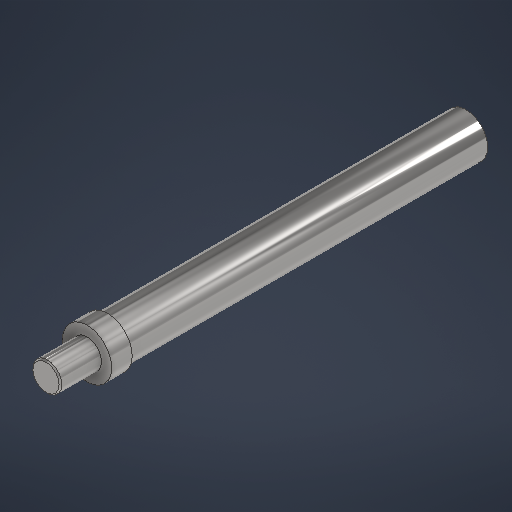
# Autodesk Inventor part: trục đai
Saved by Autodesk Inventor 2027.1 (Build 311270010, 270A)
## iProperties
Created: 2026-06-14
Part Number: trục đai
Material: Generic
Document SubType Name: Sheet Metal
Designer: MSI
Density: 1 g/cm^3
Sheet Metal Rule: Default_mm
Appearance: Steel - Polished
Author: MSI
Autodesk Inventor part; units mm, degrees
ref_plane "YZ Plane" through (0, 0, 0) normal (1, 0, 0) x (0, 1, 0)
ref_plane "XZ Plane" through (0, 0, 0) normal (0, 1, 0) x (-1, 0, 0)
ref_plane "XY Plane" through (0, 0, 0) normal (0, 0, 1) x (1, 0, 0)
sketch "Sketch1" plane through (0, 0, 0) normal (0, 0, 1) x (1, 0, 0)
  circle A0 centre (0, 0) radius 4.75
  circle A1 centre (0, 0) radius 5.4
  circle A2 centre (0, 0) radius 3.175
  dimension "d0" = 9.5
  dimension "d1" = 10.8
  dimension "d2" = 6.35
  constraints: 3 centre point, 3 coincident
  measures "d0" diameter of A0
  measures "d1" diameter of A1
  measures "d2" diameter of A2
extrude "Extrusion1" add sketch "Sketch1" along normal blind 12 contours A2
extrude "Extrusion2" add sketch "Sketch1" against normal blind 80 contours A0
extrude "Extrusion3" add sketch "Sketch1" against normal blind 1.5 contours A1
sketch "Sketch2" plane through (0, 0, 0) normal (0, 0, -1) x (-1, 0, 0)
  circle A0 centre (0, 0) radius 3.175 projected
  circle A1 centre (0, 0) radius 3.175
  constraints: 1 centre point, 1 coincident
extrude "Extrusion4" add sketch "Sketch2" along normal blind 80
chamfer "Chamfer1" distance 0.3 angle 45 1 edges at (-3.175, 0, 12)
extrude "Extrusion5" add sketch "Sketch1" along normal blind 3 contours A0 | A1
equation "\"BendRadius\" = Thickness"
equation "\"BendReliefWidth\" = Thickness"
equation "\"BendReliefDepth\" = 0.5 * Thickness"
equation "\"CornerReliefSize\" = 4 * Thickness"
equation "\"MinimumRemnant\" = 2 * Thickness"
equation "\"TransitionRadius\" = BendRadius"
equation "\"JacobiRadiusSize\" = BendRadius"
equation "\"GapSize\" = Thickness"
equation "\"Thickness\" = 0.5"
body "Solid1"
